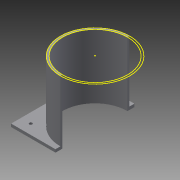
# Autodesk Inventor part: 知能ロボコン発射口ver2.5
Saved by Autodesk Inventor 2013 (Build 170138000, 138)
## iProperties
Created: 2014-06-20
Part Number: 知能ロボコン発射口ver2.5
Material: 一般
Document SubType Name: Modeling
Designer: horumo136
Density: 1 g/cm^3
Author: horumo136
Autodesk Inventor part; units mm, degrees
ref_plane "YZ Plane" through (0, 0, 0) normal (1, 0, 0) x (0, 1, 0)
ref_plane "XZ Plane" through (0, 0, 0) normal (0, 1, 0) x (-1, 0, 0)
ref_plane "XY Plane" through (0, 0, 0) normal (0, 0, 1) x (1, 0, 0)
sketch "スケッチ1" plane through (0, 0, 0) normal (0, 0, 1) x (1, 0, 0)
  circle A0 centre (0, 0) radius 35
  circle A1 centre (0, 0) radius 33
  line L0 (-45, 40) -> (45, 40)
  line L1 (45, 40) -> (45, -40)
  line L2 (45, -40) -> (-45, -40)
  line L3 (-45, -40) -> (-45, 40)
  line L4 (-45, 40) -> (45, -40) construction
  line L5 (45, 40) -> (-45, -40) construction
  dimension "d0" = 70
  dimension "d1" = 66
  dimension "d2" = 90
  dimension "d3" = 80
  constraints: 12 end point, 2 centre point, 2 coincident, 2 midpoint, 2 parallel, 1 horizontal, 1 perpendicular
  measures "d0" diameter of A0
  measures "d1" diameter of A1
  measures "d2" distance of L1.end L2.end
  measures "d3" distance of L0.end L1.end
extrude "押し出し1" add sketch "スケッチ1" along normal blind 3 contours L0 L1 L2 L3
sketch "スケッチ2" plane through (0, 0, 3) normal (0, 0, 1) x (1, 0, 0)
  circle A0 centre (0, 0) radius 35 projected
  circle A1 centre (0, 0) radius 35
  circle A2 centre (0, 0) radius 33
  dimension "d6" = 66
  constraints: 2 centre point, 2 coincident, 1 concentric
  measures "d6" diameter of A2
extrude "押し出し2" add sketch "スケッチ2" along normal blind 3 and the other way blind 3
sketch "スケッチ3" plane through (0, 0, 6) normal (0, 0, 1) x (1, 0, 0)
  circle A0 centre (0, 0) radius 33 projected
  circle A1 centre (0, 0) radius 35 projected
extrude "押し出し3" add sketch "スケッチ3" along normal blind 59
sketch "スケッチ4" plane through (0, 0, 65) normal (0, 0, 1) x (1, 0, 0)
  circle A0 centre (0, 0) radius 33 projected
  circle A1 centre (0, 0) radius 35 projected
sketch "スケッチ5" plane through (0, 0, 0) normal (0, 0, -1) x (-1, 0, 0)
  line L0 (-45, 40) -> (-35, 40)
  line L1 (-35, 40) -> (-35, 30)
  line L2 (-35, 30) -> (-45, 30)
  line L3 (-45, 30) -> (-45, 40)
  line L4 (-45, -40) -> (-35, -40)
  line L5 (-35, -40) -> (-35, -30)
  line L6 (-35, -30) -> (-45, -30)
  line L7 (-45, -30) -> (-45, -40)
  line L8 (45, -40) -> (35, -40)
  line L9 (35, -40) -> (35, -30)
  line L10 (35, -30) -> (45, -30)
  line L11 (45, -30) -> (45, -40)
  line L12 (45, 40) -> (35, 40)
  line L13 (35, 40) -> (35, 30)
  line L14 (35, 30) -> (45, 30)
  line L15 (45, 30) -> (45, 40)
  dimension "d13" = 10
  dimension "d14" = 10
  dimension "d15" = 10
  dimension "d16" = 10
  dimension "d17" = 10
  dimension "d18" = 10
  dimension "d19" = 10
  constraints: 32 end point, 8 parallel, 4 coincident, 4 horizontal, 4 perpendicular
  measures "d13" distance of L1.end L2.end
  measures "d14" distance of L0.end L1.end
  measures "d15" distance of L6.end L5.end
  measures "d16" distance of L5.end L4.end
  measures "d17" distance of L9.end L10.end
  measures "d18" distance of L8.end L9.end
  measures "d19" distance of L14.end L13.end
hole "穴1" at (35, 30, 0) at (-35, 30, 0) at (-35, -30, 0) at (35, -30, 0) direction (0, 0, 1) diameter 3 depth 8 tip angle 118
sketch "スケッチ6" plane through (0, 0, 0) normal (0, 0, -1) x (-1, 0, 0)
  circle A0 centre (-35, 30) radius 1.5 projected
  circle A1 centre (-35, -30) radius 1.5 projected
  line L0 (-45, -40) -> (45, -40) projected
  line L1 (-45, 40) -> (0, 40)
  line L2 (0, 40) -> (0, -40)
  line L3 (0, -40) -> (-45, -40)
  line L4 (-45, -40) -> (-45, 40)
  constraints: 8 end point, 2 parallel, 1 horizontal, 1 midpoint, 1 perpendicular
extrude "押し出し4" cut sketch "スケッチ6" against normal blind 65
